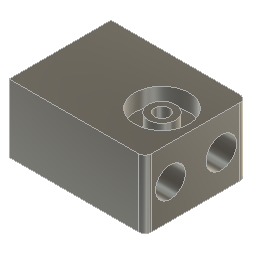
Bed Mount CR-10S (Autodesk Fusion 360 design; units mm, degrees)
Autodesk Fusion 360 part; units mm, degrees
sketch "Sketch1" plane through (0, 0, 0) normal (0, 0, 1) x (1, 0, 0)
  line L0 (0, 0) -> (40, 0)
  line L1 (40, 0) -> (40, -30)
  line L2 (40, -30) -> (0, -30)
  line L3 (0, -30) -> (0, 0)
  line L4 (30, 0) -> (30, -30) construction
  line L5 (40, -15) -> (0, -15) construction
  circle A0 centre (30, -15) radius 8
  circle A1 centre (30, -15) radius 4
  circle A2 centre (30, -15) radius 2.2
  line L6 (33.6, -12.9215) -> (30, -10.8431)
  line L7 (30, -10.8431) -> (26.4, -12.9215)
  line L8 (26.4, -12.9215) -> (26.4, -17.0785)
  line L9 (26.4, -17.0785) -> (30, -19.1569)
  line L10 (30, -19.1569) -> (33.6, -17.0785)
  line L11 (33.6, -17.0785) -> (33.6, -12.9215)
  point P0 (30, -15)
  dimension "d1" = 40
  dimension "d2" = 30
  dimension "d3" = 10
  dimension "d4" = 15
  dimension "d5" = 16
  dimension "d6" = 8
  dimension "d7" = 4.4
  dimension "d17" = 3.6
  constraint horizontal L0
  constraint vertical L1
  constraint horizontal L2
  constraint vertical L3
  constraint coincident L0.start L3.end
  constraint coincident L0 L4.start
  constraint coincident L2 L4.end
  constraint perpendicular L2 L4
  constraint coincident L1 L5.start
  constraint coincident L3 L5.end
  constraint perpendicular L3 L5
  constraint concentric A0 A1
  constraint concentric A0 A2
  constraint coincident P0 A0.centre
  constraint parallel L1 L11
  constraint midpoint L4 P0
  measures "d1" distance of L0.start L0.end
  measures "d2" distance of L0.start L2.end
  measures "d3" distance of L1 L4
  measures "d4" distance of L2 L5
  measures "d5" diameter of A0
  measures "d6" diameter of A1
  measures "d7" diameter of A2
  measures "d17" distance of P0 L11
extrude "Extrude1" add sketch "Sketch1" along normal blind 20 contours L0 L1 L2 L3
extrude "Extrude3" add sketch "Sketch1" along normal blind 15 contours A0 | A1 L6 L11 | A1 L10 L11 | A1 L6 L7 | A1 L9 L10 | A1 L7 L8 | A1 L8 L9
extrude "Extrude4" add sketch "Sketch1" along normal blind 19 contours A1 L11 | A1 L6 L7 L8 L9 L10 L11 | A1 L6 | A1 L10 | A1 L7 | A1 L9 | A1 L8 | A2
extrude "Extrude5" cut sketch "Sketch1" along normal blind 6 contours A1 L6 L7 L8 L9 L10 L11 | A1 L6 L11 | A1 L10 L11 | A1 L6 L7 | A1 L9 L10 | A1 L7 L8 | A1 L8 L9 | A2
extrude "Extrude8" cut sketch "Sketch1" along normal up to surface (12.8 mm away) from surface at 6.2 contours A2
sketch "Sketch2" plane through (40, 0, 0) normal (1, 0, 0) x (0, 1, 0)
  line L0 (-30, 0) -> (0, 0)
  line L1 (0, 0) -> (0, 20)
  line L2 (0, 20) -> (-30, 20)
  line L3 (-30, 20) -> (-30, 0)
  line L4 (-22.5, 20) -> (-22.5, 0) construction
  line L5 (-7.5, 20) -> (-7.5, 0) construction
  line L6 (-30, 10) -> (0, 10) construction
  line L7 (0, 0) -> (-30, 0) construction
  line L8 (-15, 20) -> (-15, 0) construction
  circle A0 centre (-7.5, 10) radius 2.6
  circle A1 centre (-7.5, 10) radius 4.5
  circle A2 centre (-22.5, 10) radius 2.6
  circle A3 centre (-22.5, 10) radius 4.4
  dimension "d21" = 10
  dimension "d22" = 15
  dimension "d23" = 15
  dimension "d24" = 7.5
  dimension "d25" = 5.2
  dimension "d26" = 9
  dimension "d27" = 5.2
  dimension "d28" = 8.8
  constraint coincident L2 L4.start
  constraint coincident L0 L4.end
  constraint perpendicular L0 L4
  constraint coincident L2 L5.start
  constraint coincident L0 L5.end
  constraint perpendicular L0 L5
  constraint coincident L3 L6.start
  constraint coincident L1 L6.end
  constraint perpendicular L1 L6
  constraint coincident L2 L8.start
  constraint coincident L7 L8.end
  constraint perpendicular L7 L8
  constraint midpoint L5 A0.centre
  constraint concentric A0 A1
  constraint midpoint L4 A2.centre
  constraint concentric A2 A3
  measures "d21" distance of L6 L7
  measures "d22" distance of L4 L5
  measures "d23" distance of L3 L8
  measures "d24" distance of L4 L8
  measures "d25" diameter of A0
  measures "d26" diameter of A1
  measures "d27" diameter of A2
  measures "d28" diameter of A3
extrude "Extrude6" cut sketch "Sketch2" against normal up to surface (36 mm away) contours A0 | A1 | A2 | A3
extrude "Extrude7" cut sketch "Sketch2" against normal up to surface (4 mm away) from surface at -36 contours A0 | A2
fillet "Fillet1" radius 2 2 edges at (40, 0, 10) (40, -30, 10)
